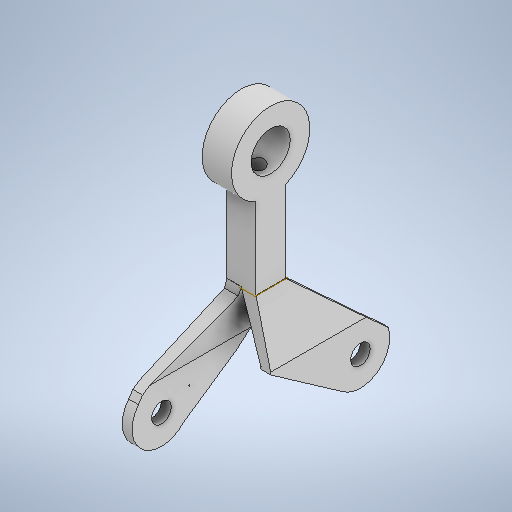
# Autodesk Inventor part: Inner_main
Saved by Autodesk Inventor 2025 (Build 290162000, 162)
## iProperties
Created: 2025-10-07
Part Number: Inner_main
Material: Типовые
Document SubType Name: Modeling
Designer: Admin
Density: 1 g/cm^3
Appearance: По умолчанию
Author: Admin
Autodesk Inventor part; units mm, degrees
ref_plane "YZ Plane" through (0, 0, 0) normal (1, 0, 0) x (0, 1, 0)
ref_plane "XZ Plane" through (0, 0, 0) normal (0, 1, 0) x (-1, 0, 0)
ref_plane "XY Plane" through (0, 0, 0) normal (0, 0, 1) x (1, 0, 0)
sketch "Эскиз1" plane through (0, 0, 0) normal (1, 0, 0) x (0, 1, 0)
  circle A0 centre (-11.8316, 3.105) radius 10
  line L0 (-11.8316, 3.105) -> (-11.8316, -16.895)
  line L1 (-11.8316, -16.895) -> (-11.8316, 23.105)
  line L2 (108.1684, -16.895) -> (108.1684, 23.105)
  line L3 (-11.8316, 3.105) -> (-117.0772, 41.4113)
  line L4 (-11.8316, 3.105) -> (-102.8044, 3.105)
  line L5 (-11.8316, 3.105) -> (-117.0772, -35.2012)
  circle A1 centre (-117.0772, 41.4113) radius 15
  circle A2 centre (-117.0772, -35.2012) radius 15
  line L6 (-11.8316, 3.105) -> (-71.8316, 3.105)
  line L7 (-71.8316, 3.105) -> (-104.4836, 49.56)
  line L8 (-71.8316, 3.105) -> (-104.8037, -43.8244)
  line L9 (-11.8316, 23.105) -> (-85.8891, 23.105)
  line L10 (-11.8316, -16.895) -> (-85.8834, -16.895)
  line L11 (-71.8316, 3.105) -> (-108.4958, 3.105)
  line L12 (-108.4958, 3.105) -> (-129.0093, 32.3215)
  line L13 (-108.4958, 3.105) -> (-129.3507, -26.578)
  circle A3 centre (-117.0772, 41.4113) radius 5
  circle A4 centre (-117.0772, -35.2012) radius 5
  point P0 (0, 0)
  dimension "d0" = 20
  dimension "d1" = 20
  dimension "d2" = 40
  dimension "d3" = 120
  dimension "d4" = 40
  dimension "d5" = 112
  dimension "d6" = 20
  dimension "d7" = 112
  dimension "d8" = 20
  dimension "d9" = 30
  dimension "d10" = 30
  dimension "d11" = 60
  dimension "d30" = 10
  dimension "d31" = 10
  constraints: 28 end point, 5 centre point, 5 point on line, 4 coincident, 4 point on circle, 2 horizontal, 2 parallel, 2 tangent, 1 vertical
  measures "d0" diameter of A0
  measures "d1" distance of L0.start L0.end
  measures "d2" distance of L0.end L1.end
  measures "d3" distance of L0.end L2.start
  measures "d4" distance of L2.start L2.end
  measures "d5" distance of L0.start L3.end
  measures "d6" angle of L4 L3
  measures "d7" distance of L0.start L5.end
  measures "d8" angle of L5 L4
  measures "d9" diameter of A1
  measures "d10" diameter of A2
  measures "d11" distance of L0.start L6.end
  measures "d30" diameter of A3
  measures "d31" diameter of A4
extrude "Выдавливание1" add sketch "Эскиз1" along normal blind 5 contours A1 | A3
ref_plane "РабПлоскость2" through (30, -117.0772, 41.4113) normal (1, 0, 0) x (0, 0, -1)
ref_plane "РабПлоскость3" through (0, -11.8316, 3.105) normal (0, 0, -1) x (-1, 0, 0)
sketch "Эскиз3" plane through (0, -11.8316, 3.105) normal (0, 0, -1) x (-1, 0, 0)
  point P0 (0, 11.8316)
extrude "Выдавливание3" cut sketch "Эскиз1" along normal blind 10 contours A3
sketch "Эскиз4" plane through (0, -11.8316, 3.105) normal (0, 0, -1) x (-1, 0, 0)
  line L0 (0, 0) -> (-30, 0)
  line L1 (-30, 0) -> (-30, -122.0926)
  line L2 (-15, 0) -> (-15, -60)
  line L3 (-15, -60) -> (-22.5, -60)
  line L4 (-15, -60) -> (-7.5, -60)
  line L5 (-7.5, -60) -> (-7.5, 0)
  line L6 (-22.5, -60) -> (-22.5, 0)
  line L7 (-7.5, -60) -> (0, -90.2456)
  line L8 (-5, -90.2456) -> (-5, -120.2456) projected
  line L9 (0, -90.2456) -> (-5, -90.2456)
  line L10 (-5, -90.2456) -> (-15, -60)
  line L11 (0, -90.2456) -> (0, -100.2456)
  line L12 (0, -90.2456) -> (0, -120.2456) projected
  line L13 (0, -100.2456) -> (-5, -100.2456)
  line L14 (-5, -90.2456) -> (-5, -100.2456)
  point P0 (0, 11.8316)
  dimension "d34" = 30
  dimension "d35" = 60
  dimension "d36" = 7.5
  dimension "d37" = 7.5
  dimension "d40" = 10
  constraints: 26 end point, 6 perpendicular, 4 point on line, 2 horizontal, 1 collinear, 1 midpoint, 1 vertical
  measures "d34" distance of L0.start L0.end
  measures "d35" distance of L2.start L2.end
  measures "d36" distance of L2.end L3.end
  measures "d37" distance of L2.end L4.end
  measures "d40" distance of L7.end L11.end
extrude "Выдавливание4" add sketch "Эскиз4" along normal mid plane 15 contours L5 L4 L2 L0 | L2 L3 L6 L0
extrude "Выдавливание5" add sketch "Эскиз4" against normal blind 50 contours L7 L9 L10 L4 | L11 L13 L8 L9
sketch "Эскиз5" plane through (0, 0, 0) normal (-1, 0, 0) x (0, 0, 1)
  arc A0 (27.2692, -112.0772) -> (53.105, -107.6827) centre (41.4113, -117.0772) ccw projected
  line L0 (53.105, -107.6827) -> (53.105, -71.8316)
  line L1 (3.105, -102.0772) -> (3.105, -71.8316) projected
  line L2 (53.105, -71.8316) -> (3.105, -71.8316)
  line L3 (3.105, -71.8316) -> (51.0193, -104.5042)
  line L4 (51.0193, -104.5042) -> (53.105, -107.6827)
  line L5 (3.105, -102.0772) -> (3.105, -112.0772) projected
  line L6 (3.105, -108.5643) -> (3.105, -112.0772)
  line L7 (3.105, -112.0772) -> (8.2567, -112.0772)
  line L8 (8.2567, -112.0772) -> (3.105, -108.5643)
  line L9 (8.2567, -112.0772) -> (26.8337, -112.0772)
  line L10 (26.8337, -112.0772) -> (32.327, -128.4906)
  line L11 (32.327, -128.4906) -> (8.2567, -112.0772)
  line L12 (10.4648, -71.8316) -> (10.4648, -76.8502)
  point P0 (0, 0)
  point P1 (30.1949, -127.0368)
  point P2 (27.0537, -112.7345)
  constraints: 22 end point, 4 point on line, 2 parallel, 2 perpendicular, 2 vertical
extrude "Выдавливание6" cut sketch "Эскиз5" against normal blind 50 contours L4 L3 L12 L2 L0 | L7 L5 L8
extrude "Выдавливание7" add sketch "Эскиз5" against normal blind 5 contours A0 L11 L9 L10
extrude "Выдавливание8" add sketch "Эскиз4" along normal blind 7.5 contours L7 L9 L10 L4
sketch "Эскиз6" plane through (30, -117.0772, 41.4113) normal (1, 0, 0) x (0, 0, -1)
  circle A0 centre (38.306, 105.2458) radius 10
  line L0 (38.306, 105.2458) -> (58.306, 105.2458)
  line L1 (58.306, 105.2458) -> (18.306, 105.2458)
  line L2 (58.306, 225.2458) -> (18.306, 225.2458)
  line L3 (38.306, 105.2458) -> (-0.0002, 0.0003)
  line L4 (38.306, 105.2458) -> (38.306, 14.273)
  line L5 (38.306, 105.2458) -> (76.6123, 0.0003)
  circle A1 centre (-0.0002, 0.0003) radius 15
  circle A2 centre (76.6123, 0.0003) radius 15
  line L6 (38.306, 105.2458) -> (38.306, 45.2458)
  line L7 (38.306, 45.2458) -> (-8.1489, 12.5939)
  line L8 (38.306, 45.2458) -> (85.2355, 12.2738)
  line L9 (18.306, 105.2458) -> (18.306, 31.1884)
  line L10 (58.306, 105.2458) -> (58.306, 31.1941)
  line L11 (38.306, 45.2458) -> (38.306, 8.5816)
  line L12 (38.306, 8.5816) -> (9.0896, -11.9318)
  line L13 (38.306, 8.5816) -> (67.9891, -12.2733)
  circle A3 centre (-0.0002, 0.0003) radius 5
  circle A4 centre (76.6123, 0.0003) radius 5
  point P0 (41.4113, 117.0772)
  point P1 (41.4111, 117.0775)
  dimension "d49" = 20
  dimension "d50" = 20
  dimension "d51" = 40
  dimension "d52" = 120
  dimension "d53" = 40
  dimension "d54" = 112
  dimension "d55" = 20
  dimension "d56" = 112
  dimension "d57" = 20
  dimension "d58" = 30
  dimension "d59" = 30
  dimension "d60" = 60
  dimension "d61" = 10
  dimension "d62" = 10
  constraints: 28 end point, 5 centre point, 5 point on line, 4 coincident, 4 point on circle, 2 parallel, 2 tangent
  measures "d49" diameter of A0
  measures "d50" distance of L0.start L0.end
  measures "d51" distance of L0.end L1.end
  measures "d52" distance of L0.end L2.start
  measures "d53" distance of L2.start L2.end
  measures "d54" distance of L0.start L3.end
  measures "d55" angle of L4 L3
  measures "d56" distance of L0.start L5.end
  measures "d57" angle of L5 L4
  measures "d58" diameter of A1
  measures "d59" diameter of A2
  measures "d60" distance of L0.start L6.end
  measures "d61" diameter of A3
  measures "d62" diameter of A4
extrude "Выдавливание9" add sketch "Эскиз6" against normal blind 5 contours A2
sketch "Эскиз7" plane through (0, -11.8316, 3.105) normal (0, 0, -1) x (-1, 0, 0)
  line L0 (-15, -60) -> (-13.3407, -65.0186) projected
  line L1 (-25, -120.2453) -> (-25, -90.2453) projected
  line L2 (-15, -60) -> (-25, -90.2453)
  line L3 (-30, -90.2453) -> (-30, -120.2453) projected
  line L4 (-25, -90.2453) -> (-30, -90.2453)
  line L5 (-22.5, 0) -> (-22.5, -60) projected
  line L6 (-30, -90.2453) -> (-22.5, -60)
  line L7 (-22.5, -60) -> (-15, -60)
  line L8 (-25, -90.2453) -> (-25, -100.2453)
  line L9 (-25, -100.2453) -> (-30, -100.2453)
  line L10 (-30, -100.2453) -> (-30, -90.2453)
  point P0 (0, 11.8316)
  dimension "d65" = 10
  constraints: 14 end point, 5 perpendicular
  measures "d65" distance of L1.end L8.end
extrude "Выдавливание10" add sketch "Эскиз7" along normal blind 60 and the other way blind 7.5
sketch "Эскиз8" plane through (30, -117.0772, 41.4113) normal (1, 0, 0) x (0, 0, -1)
  arc A0 (62.4702, 5.0003) -> (90.7544, 5.0003) centre (76.6123, 0.0003) ccw projected
  line L0 (38.3063, 15) -> (38.3063, 8.5129) projected
  line L1 (68.2738, -12.4685) -> (38.3063, 8.5129)
  line L2 (38.3063, 8.5129) -> (33.2066, 5.0003)
  line L3 (30.8063, 5.0003) -> (62.4702, 5.0003) projected
  line L4 (33.2066, 5.0003) -> (43.3234, 5.0003)
  line L5 (43.3234, 5.0003) -> (66.6625, 5.0003)
  line L6 (66.6625, 5.0003) -> (68.2738, -12.4685)
  line L7 (45.8063, 45.2456) -> (98.3063, 45.2456) projected
  line L8 (90.6076, 5.0003) -> (45.8063, 45.2456)
  line L9 (45.8063, 45.2456) -> (99.0886, 48.0677)
  line L10 (99.0886, 48.0677) -> (105.849, 29.5221)
  line L11 (105.849, 29.5221) -> (100.0021, 2.5717)
  line L12 (100.0021, 2.5717) -> (90.6076, 5.0003)
  point P0 (41.4113, 117.0772)
  constraints: 20 end point, 4 point on line, 1 horizontal, 1 point on circle
extrude "Выдавливание11" cut sketch "Эскиз8" against normal blind 60 contours L1 L3 L5 L6 | L8 L9 L10 L11 L12
extrude "Выдавливание12" add sketch "Эскиз8" against normal blind 5 contours L1 L3 L5 L6
sketch "Эскиз9" plane through (0, 0, 0) normal (-1, 0, 0) x (0, 0, 1)
  line L0 (3.105, -108.5643) -> (3.105, -102.0772) projected
  line L1 (3.105, -108.5643) -> (-4.395, -102.0772)
  line L2 (3.105, -102.0772) -> (47.4601, -102.0772) projected
  line L3 (-4.395, -102.0772) -> (3.105, -102.0772)
  line L4 (3.105, -102.0772) -> (3.105, -108.5643)
  point P0 (0, 0)
  constraints: 6 end point, 1 collinear, 1 perpendicular
extrude "Выдавливание13" add sketch "Эскиз9" against normal blind 5
sketch "Эскиз10" plane through (30, -117.0772, 41.4113) normal (1, 0, 0) x (0, 0, -1)
  line L0 (38.3063, 8.5129) -> (45.8063, 15) projected
  line L1 (43.3234, 5.0003) -> (38.3063, 8.5129)
  line L2 (38.3063, 8.5129) -> (30.8063, 13.764)
  line L3 (30.8063, 5.0003) -> (43.3234, 5.0003) projected
  line L4 (30.8063, 13.764) -> (30.8063, 5.0003)
  line L5 (30.8063, 5.0003) -> (43.3234, 5.0003)
  point P0 (41.4113, 117.0772)
  constraints: 8 end point, 2 perpendicular, 1 point on line
extrude "Выдавливание14" cut sketch "Эскиз10" against normal blind 5
sketch "Эскиз11" plane through (22.5, -11.8316, 10.605) normal (1, 0, 0) x (0, 0, -1)
  line L0 (0, 0) -> (15, 0) projected
  circle A0 centre (7.5, 0) radius 10
  circle A1 centre (7.5, 0) radius 20
  point P0 (10.605, 11.8316)
  dimension "d78" = 20
  dimension "d79" = 40
  constraints: 2 centre point, 1 coincident, 1 midpoint
  measures "d78" diameter of A0
  measures "d79" diameter of A1
extrude "Выдавливание15" add sketch "Эскиз11" against normal blind 15
extrude "Выдавливание16" cut sketch "Эскиз11" against normal blind 15 contours A0
ref_plane "РабПлоскость4" through (15, -71.8316, 10.605) normal (0, 1, 0) x (1, 0, 0)
sketch "Эскиз12" plane through (15, -71.8316, 10.605) normal (0, 1, 0) x (1, 0, 0)
  line L0 (0, 0.1403) -> (0, 15) projected
  circle A0 centre (0, 7.5701) radius 4
  point P0 (-15, 10.605)
  dimension "d84" = 8
  constraints: 1 centre point, 1 midpoint
  measures "d84" diameter of A0
extrude "Выдавливание17" cut sketch "Эскиз12" along normal blind 60 and the other way blind 30
